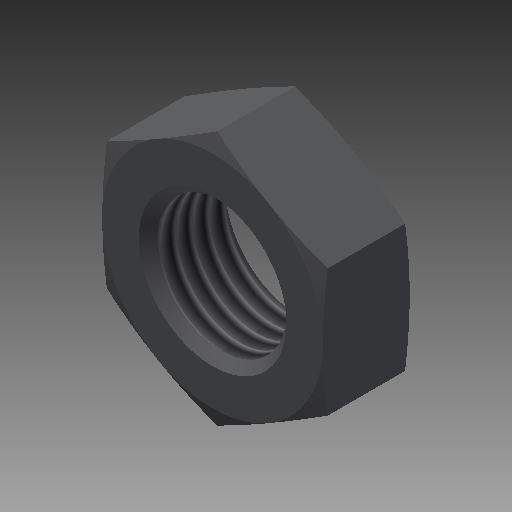
# Autodesk Inventor part: D-801
Saved by Autodesk Inventor 2017 (Build 210142000, 142)
## iProperties
Category: PARTsolutions
Company: BIMBA
Created: 2017-01-31
Part Number: D-801
Catalog Web Link: www.cadenas.de
Description: Mounting Nut for Original Line Cylinders-
Vendor: BIMBA
Document SubType Name: Modeling
Designer: psAdmin
Manufacturer: BIMBA
Mass: 0.659017 g
Surface Area: 6.36957 cm^2
Volume: 0.659017 cm^3
Density: 1 g/cm^3
Material: Generic
Appearance: PSOLRGB-191-191-191
PSOL_IDENT_0: {$CADENAS_DATA\23d-libs\bimba\bimba\bimba_imperial\bimba_full_line\original_line_cylinders\accessori
PSOL_IDENT_1: es\mounting_nut.prj},190 {VTYP=3D},{NB=D-801},{LINA=D-801},{NN=Mounting Nut for Original Line Cylind
PSOL_IDENT_2: ers},{DATE=09.11.2016 07:55:10},{GEOMDATE=10.11.2011 00:00:00},{VERSION=},{LINEID=300},{LINESUBID=-1
PSOL_IDENT_3: },{WBVAR=MAT}  {NB=D-801},{LINA=D-801},{KT=DUMMY},{PN=D-801},{PN1=D-801},{C=3/8-24},{TH=UNF},{MAT=},
PSOL_IDENT_4: {MAT1='','Zinc-Plated Carbon Steel', '-SS', 'Stainless Steel'},{A=0.56},{A1=0.56000000},{B=0.22},{B1=
PSOL_IDENT_5: 0.22000000},{NDM=0.37500000},{PITCH=0.0417},{DIA=-},{DIA2=-},{DIA3=-},{DIA1=0},{DIA4=0.00000000},{DI
PSOL_IDENT_6: A5=0.00000000},{T=-},{T2=-},{T3=-},{T1=0},{T4=0.00000000},{T5=0.00000000},{COLOR=0.75,0.75,0.75,0.00
PSOL_IDENT_7: },{TT=0.05000000},{TO=0.15000000},{PRA=1}
NN: Mounting Nut for Original Line Cylinders
NB: D-801
NBSYN: $PN.
LINA: D-801
PN: D-801
C: 3/8-24
MAT: Zinc-Plated Carbon Steel
A: 0.56
B: 0.22
DIA: -
T: -
SUPPLIER: BIMBA
ARTICLENO: D-801
BOMINFO: D-801
CREATOR: CADENAS GmbH
Title: D-801
Author: Cadenas PARTsolutions
Autodesk Inventor part; units mm, degrees
sketch "Sketch_8" plane through (0, 0, 0) normal (1, 0, 0) x (0, 1, 0)
  line L0 (0, -5.588) -> (0, 0)
  line L1 (0, 0) -> (7.112, 0)
  line L2 (7.112, 0) -> (8.5344, -0.3811)
  line L3 (8.5344, -0.3811) -> (8.5344, -5.2069)
  line L4 (8.5344, -5.2069) -> (7.112, -5.588)
  line L5 (7.112, -5.588) -> (0, -5.588)
  line L6 (0, -5.588) -> (0, 0)
  constraints: 14 end point
sketch "Sketch_10" plane through (0, 0, 0) normal (0, 0, 1) x (1, 0, 0)
  line L0 (-14.224, -14.224) -> (14.224, -14.224)
  line L1 (14.224, -14.224) -> (14.224, 14.224)
  line L2 (14.224, 14.224) -> (-14.224, 14.224)
  line L3 (-14.224, 14.224) -> (-14.224, -14.224)
  line L4 (-7.112, -4.1061) -> (0, -8.2122)
  line L5 (0, -8.2122) -> (7.112, -4.1061)
  line L6 (7.112, -4.1061) -> (7.112, 4.1061)
  line L7 (7.112, 4.1061) -> (0, 8.2122)
  line L8 (0, 8.2122) -> (-7.112, 4.1061)
  line L9 (-7.112, 4.1061) -> (-7.112, -4.1061)
  constraints: 20 end point
revolve "Revolution1" add sketch "Sketch_8" angle 360 about axis through (0, 0, -5.588) along (0, 0, -1)
extrude "Extrusion1" cut sketch "Sketch_10" against normal blind 5.588
sketch "Sketch_11" plane through (0, 0, 0) normal (1, 0, 0) x (0, 1, 0)
  line L0 (0, -5.588) -> (0, 0)
  line L1 (0, 0) -> (4.7625, 0)
  line L2 (4.7625, 0) -> (4.1897, -0.5728)
  line L3 (4.1897, -0.5728) -> (4.1897, -5.0152)
  line L4 (4.1897, -5.0152) -> (4.7625, -5.588)
  line L5 (4.7625, -5.588) -> (0, -5.588)
  line L6 (0, -5.588) -> (0, 0)
  constraints: 14 end point
revolve "Revolution2" cut sketch "Sketch_11" angle 360 about axis through (0, 0, -5.588) along (0, 0, -1)
thread "Thread1" size "3/8-24 UNF" class "2B" standard "ANSI Unified Screw Threads" full length
ref_plane "NUT_XY" through (0, 0, 0) normal (0, 0, 1) x (1, 0, 0)
ref_plane "NUT_YZ" through (0, 0, 0) normal (1, 0, 0) x (0, 1, 0)
ref_plane "NUT_ZX" through (0, 0, 0) normal (0, 1, 0) x (0, 0, 1)
ref_plane "a1_XY" through (-7.112, 7.112, 0) normal (0, 0, 1) x (1, 0, 0)
ref_plane "a1_YZ" through (-7.112, 7.112, 0) normal (1, 0, 0) x (0, 1, 0)
ref_plane "a1_ZX" through (-7.112, 7.112, 0) normal (0, 1, 0) x (0, 0, 1)
ref_plane "a2_XY" through (7.112, 7.112, 0) normal (0, 0, 1) x (1, 0, 0)
ref_plane "a2_YZ" through (7.112, 7.112, 0) normal (1, 0, 0) x (0, 1, 0)
ref_plane "a2_ZX" through (7.112, 7.112, 0) normal (0, 1, 0) x (0, 0, 1)
ref_plane "b1_XY" through (0, 7.112, 0) normal (1, 0, 0) x (0, 0, -1)
ref_plane "b1_YZ" through (0, 7.112, 0) normal (0, 0, -1) x (0, 1, 0)
ref_plane "b1_ZX" through (0, 7.112, 0) normal (0, 1, 0) x (1, 0, 0)
ref_plane "b2_XY" through (0, 7.112, -5.588) normal (1, 0, 0) x (0, 0, -1)
ref_plane "b2_YZ" through (0, 7.112, -5.588) normal (0, 0, -1) x (0, 1, 0)
ref_plane "b2_ZX" through (0, 7.112, -5.588) normal (0, 1, 0) x (1, 0, 0)
ref_plane "e_XY" through (0, 0, -5.588) normal (1, 0, 0) x (0, 0, -1)
ref_plane "e_YZ" through (0, 0, -5.588) normal (0, 0, -1) x (0, 1, 0)
ref_plane "e_ZX" through (0, 0, -5.588) normal (0, 1, 0) x (1, 0, 0)
ref_plane "ol1_XY" through (0, 0, -7.112) normal (0, 1, 0) x (1, 0, 0)
ref_plane "ol1_YZ" through (0, 0, -7.112) normal (1, 0, 0) x (0, 0, -1)
ref_plane "ol1_ZX" through (0, 0, -7.112) normal (0, 0, -1) x (0, 1, 0)
ref_plane "ol2_XY" through (5.588, 0, -7.112) normal (0, 1, 0) x (1, 0, 0)
ref_plane "ol2_YZ" through (5.588, 0, -7.112) normal (1, 0, 0) x (0, 0, -1)
ref_plane "ol2_ZX" through (5.588, 0, -7.112) normal (0, 0, -1) x (0, 1, 0)
ref_plane "th1_XY" through (0, 4.7625, -5.588) normal (1, 0, 0) x (0, 0, -1)
ref_plane "th1_YZ" through (0, 4.7625, -5.588) normal (0, 0, -1) x (0, 1, 0)
ref_plane "th1_ZX" through (0, 4.7625, -5.588) normal (0, 1, 0) x (1, 0, 0)
ref_plane "th2_XY" through (0, -4.7625, -5.588) normal (1, 0, 0) x (0, 0, -1)
ref_plane "th2_YZ" through (0, -4.7625, -5.588) normal (0, 0, -1) x (0, 1, 0)
ref_plane "th2_ZX" through (0, -4.7625, -5.588) normal (0, 1, 0) x (1, 0, 0)
body "Solid1"
